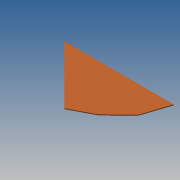
# Autodesk Inventor part: wrapAround
Saved by Autodesk Inventor 2013 (Build 170138000, 138)
## iProperties
Created: 2014-01-02
Part Number: wrapAround
Material: Wood (Cherry)
Document SubType Name: Modeling
Designer: ddeboer
Mass: 218941 g
Surface Area: 235270 cm^2
Volume: 437882 cm^3
Density: 0.5 g/cm^3
Author: ddeboer
Autodesk Inventor part; units mm, degrees
ref_plane "YZ Plane" through (0, 0, 0) normal (1, 0, 0) x (0, 1, 0)
ref_plane "XZ Plane" through (0, 0, 0) normal (0, 1, 0) x (-1, 0, 0)
ref_plane "XY Plane" through (0, 0, 0) normal (0, 0, 1) x (1, 0, 0)
sketch "Sketch1" plane through (0, 0, 0) normal (0, 1, 0) x (-1, 0, 0)
  line L0 (0, 0) -> (4876.8, 0)
  line L1 (4876.8, 0) -> (395.816, 1200.676) construction
  line L2 (4876.8, 0) -> (1294.8012, 2068.068) construction
  line L3 (4876.8, 0) -> (2292.6415, 2584.1585) construction
  line L4 (4876.8, 0) -> (3221.736, 2866.6549) construction
  line L5 (4876.8, 0) -> (4071.3531, 3005.9689) construction
  line L6 (4876.8, 0) -> (7988.808, 0) construction
  line L7 (2292.6415, 2584.1585) -> (1294.8012, 2068.068)
  line L8 (1294.8012, 2068.068) -> (395.816, 1200.676)
  line L9 (395.816, 1200.676) -> (0, 0)
  line L10 (2292.6415, 2584.1585) -> (4876.8, 0)
  dimension "d0" = 4876.8
  dimension "d8" = 4639.056
  dimension "d9" = 15
  dimension "d10" = 4136.136
  dimension "d11" = 30
  dimension "d12" = 3654.552
  dimension "d13" = 45
  dimension "d14" = 3310.128
  dimension "d15" = 60
  dimension "d18" = 3112.008
  dimension "d19" = 105
  constraints: 22 end point, 2 horizontal, 1 collinear, 1 equal length
  measures "d0" distance of L0.start L0.end
  measures "d8" distance of L0.end L1.end
  measures "d9" angle of L0 L1
  measures "d10" distance of L0.end L2.end
  measures "d11" angle of L0 L2
  measures "d12" distance of L0.end L3.end
  measures "d13" angle of L0 L3
  measures "d14" distance of L0.end L4.end
  measures "d15" angle of L0 L4
  measures "d18" distance of L0.end L5.end
  measures "d19" angle of L6 L5
extrude "Extrusion1" add sketch "Sketch1" along normal blind 38.1
body "Solid1"
